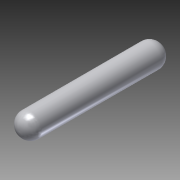
# Autodesk Inventor part: Air Tank
Saved by Autodesk Inventor 2013 (Build 170138000, 138)
## iProperties
Created: 2013-02-19
Part Number: Air Tank
Material: Generic
Document SubType Name: Modeling
Designer: zagerst
Density: 1 g/cm^3
Author: zagerst
Autodesk Inventor part; units mm, degrees
ref_plane "YZ Plane" through (0, 0, 0) normal (1, 0, 0) x (0, 1, 0)
ref_plane "XZ Plane" through (0, 0, 0) normal (0, 1, 0) x (-1, 0, 0)
ref_plane "XY Plane" through (0, 0, 0) normal (0, 0, 1) x (1, 0, 0)
sketch "Sketch1" plane through (0, 0, 0) normal (0, 0, 1) x (1, 0, 0)
  circle A0 centre (0, 0) radius 25.4
  dimension "d0" = 50.8
  constraints: 1 centre point, 1 coincident
  measures "d0" diameter of A0
extrude "Extrusion1" add sketch "Sketch1" along normal blind 304.8
fillet "Fillet1" radius 24.13 1 edges at (-25.4, 0, 304.8)
fillet "Fillet2" radius 24.13 1 edges at (-25.4, 0, 0)
body "Solid1"
